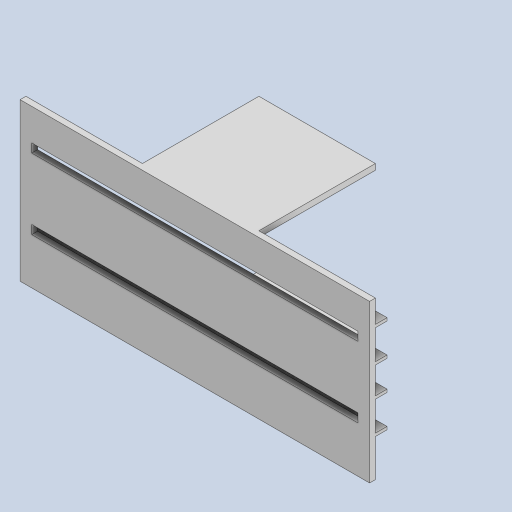
# Autodesk Inventor part: hand-box
Saved by Autodesk Inventor 2023 (Build 270158000, 158)
## iProperties
Created: 2024-11-28
Part Number: hand-box
Material: Generic
Document SubType Name: Modeling
Designer: kiyo
Density: 1 g/cm^3
Appearance: Default
Author: kiyo
Autodesk Inventor part; units mm, degrees
ref_plane "YZ Plane" through (0, 0, 0) normal (1, 0, 0) x (0, 1, 0)
ref_plane "XZ Plane" through (0, 0, 0) normal (0, 1, 0) x (-1, 0, 0)
ref_plane "XY Plane" through (0, 0, 0) normal (0, 0, 1) x (1, 0, 0)
sketch "スケッチ1" plane through (0, 0, 0) normal (1, 0, 0) x (0, 1, 0)
  line L0 (60, -16.042) -> (-60, -16.042)
  line L1 (-60, -16.042) -> (-60, 16.042)
  line L2 (-60, 16.042) -> (60, 16.042)
  line L3 (60, 16.042) -> (60, -16.042)
  line L4 (60, -16.042) -> (-60, 16.042) construction
  line L5 (-60, -16.042) -> (60, 16.042) construction
  line L6 (-56, 13.625) -> (56, 13.625)
  line L7 (56, 13.625) -> (56, 10.625)
  line L8 (56, 10.625) -> (-56, 10.625)
  line L9 (-56, 10.625) -> (-56, 13.625)
  line L10 (-56, -10.625) -> (56, -10.625)
  line L11 (56, -10.625) -> (56, -13.625)
  line L12 (56, -13.625) -> (-56, -13.625)
  line L13 (-56, -13.625) -> (-56, -10.625)
  line L14 (60, -16.042) -> (-60, -16.042)
  line L15 (-60, -16.042) -> (-60, -29.5)
  line L16 (-60, -29.5) -> (60, -29.5)
  line L17 (60, -29.5) -> (60, -16.042)
  line L18 (-60, 16.042) -> (60, 16.042)
  line L19 (60, 16.042) -> (60, 24.5)
  line L20 (60, 24.5) -> (-60, 24.5)
  line L21 (-60, 24.5) -> (-60, 16.042)
  point P0 (0, 0)
  point P1 (0, 0)
  point P2 (56, 12.125)
  point P3 (56, -12.125)
  point P4 (0, 0)
  dimension "d1" = 120
  dimension "d3" = 12.125
  dimension "d6" = 3
  dimension "d11" = 12.125
  dimension "d15" = 2.417
  dimension "d26" = 4
  dimension "d27" = 4
  dimension "d41" = 29.5
  dimension "d53" = 54
  constraints: 44 end point, 10 parallel, 6 midpoint, 5 horizontal, 5 perpendicular, 3 collinear, 2 point on line
  measures "d1" distance of L1.end L2.end
  measures "d3" vertical distance of point (56, -12.125) point (0, 0)
  measures "d6" distance of L8.end L6.start
  measures "d11" vertical distance of point (0, 0) point (56, 12.125)
  measures "d15" distance between parallel lines of L2 L6
  measures "d26" distance between parallel lines of L3 L7
  measures "d27" distance between parallel lines of L1 L9
  measures "d41" distance from line of L16 point (0, 0)
  measures "d53" distance between parallel lines of L16 L20
extrude "押し出し1" add sketch "スケッチ1" along normal blind 2
sketch "スケッチ3" plane through (0, 0, 0) normal (-1, 0, 0) x (0, 0, 1)
  line L0 (-29.5, 60) -> (24.5, 60) projected
  line L1 (5.575, 60) -> (4.575, 60)
  line L2 (4.575, 60) -> (4.575, 7)
  line L3 (4.575, 7) -> (5.575, 7)
  line L4 (5.575, 7) -> (5.575, 60)
  line L5 (16.675, 60) -> (15.675, 60)
  line L6 (15.675, 60) -> (15.675, 0)
  line L7 (15.675, 0) -> (16.675, 0)
  line L8 (16.675, 0) -> (16.675, 60)
  line L9 (0, 0) -> (4.575, 0)
  line L10 (0, 0) -> (0, 19.0491)
  line L11 (5.575, -60) -> (4.575, -60)
  line L12 (4.575, -60) -> (4.575, -7)
  line L13 (4.575, -7) -> (5.575, -7)
  line L14 (5.575, -7) -> (5.575, -60)
  line L15 (16.675, -60) -> (15.675, -60)
  line L16 (15.675, -60) -> (15.675, 0)
  line L17 (16.675, 0) -> (16.675, -60)
  line L18 (-5.575, 60) -> (-4.575, 60)
  line L19 (-4.575, 60) -> (-4.575, 7)
  line L20 (-4.575, 7) -> (-5.575, 7)
  line L21 (-5.575, 7) -> (-5.575, 60)
  line L22 (-16.675, 60) -> (-15.675, 60)
  line L23 (-15.675, 60) -> (-15.675, 0)
  line L24 (-15.675, 0) -> (-16.675, 0)
  line L25 (-16.675, 0) -> (-16.675, 60)
  line L26 (-5.575, -60) -> (-4.575, -60)
  line L27 (-4.575, -60) -> (-4.575, -7)
  line L28 (-4.575, -7) -> (-5.575, -7)
  line L29 (-5.575, -7) -> (-5.575, -60)
  line L30 (-16.675, -60) -> (-15.675, -60)
  line L31 (-15.675, -60) -> (-15.675, 0)
  line L32 (-16.675, 0) -> (-16.675, -60)
  point P0 (-15.675, 60)
  point P1 (-16.675, 60)
  point P2 (15.675, 60)
  point P3 (0, 9.5245)
  dimension "d31" = 1
  dimension "d33" = 1
  dimension "d34" = 60
  dimension "d35" = 10.1
  dimension "d36" = 7
  dimension "d61" = 5.575
  constraints: 64 end point, 20 symmetric about line, 4 parallel, 3 horizontal, 2 perpendicular, 1 midpoint, 1 point on line, 1 vertical
  measures "d31" distance of L2.end L3.end
  measures "d33" distance of L6.end L7.end
  measures "d34" distance of L7.end L5.start
  measures "d35" distance between parallel lines of L6 L4
  measures "d36" distance from line of L9.start L3
  measures "d61" distance between parallel lines of L4 L10
extrude "押し出し4" add sketch "スケッチ3" along normal blind 4
sketch "スケッチ5" plane through (0, 0, 0) normal (-1, 0, 0) x (0, 0, 1)
  line L0 (-29.5, -60) -> (-29.5, 60) projected
  line L1 (-29.5, 20) -> (-27.5, 20)
  line L2 (-27.5, 20) -> (-27.5, -20)
  line L3 (-27.5, -20) -> (-29.5, -20)
  line L4 (-29.5, -20) -> (-29.5, 60)
  line L5 (24.5, 60) -> (24.5, -60) projected
  line L6 (24.5, 20) -> (22.5, 20)
  line L7 (22.5, 20) -> (22.5, -20)
  line L8 (22.5, -20) -> (24.5, -20)
  line L9 (24.5, -20) -> (24.5, 20)
  point P0 (0, 0)
  point P1 (-29.5, -20)
  dimension "d42" = 2
  dimension "d55" = 20
  dimension "d56" = 20
  dimension "d57" = 2
  constraints: 16 end point, 4 parallel, 2 collinear, 2 horizontal, 2 perpendicular, 2 point on line
  measures "d42" distance between parallel lines of L0 L2
  measures "d55" distance from line of point (0, 0) L3
  measures "d56" distance from line of L1 point (0, 0)
  measures "d57" distance of L7.end L8.end
extrude "押し出し5" add sketch "スケッチ5" along normal blind 40
sketch "スケッチ6" plane through (2, -60, -29.5) normal (0, 0, -1) x (-1, 0, 0)
  circle A0 centre (20.75, 67) radius 1.6
  circle A1 centre (20.75, 53) radius 1.6
  line L0 (0, 0) -> (0, 120) projected
  point P0 (2, 60)
  point P1 (0, 60)
  dimension "d45" = 3.2
  dimension "d46" = 3.2
  dimension "d47" = 14
  dimension "d48" = 7
  dimension "d49" = 20.75
  dimension "d50" = 20.75
  constraints: 2 centre point, 1 midpoint
  measures "d45" diameter of A0
  measures "d46" diameter of A1
  measures "d47" distance of A0.centre A1.centre
  measures "d48" vertical distance of point (0, 60) A0.centre
  measures "d49" distance from line of L0 A0.centre
  measures "d50" distance from line of L0 A1.centre
extrude "押し出し6" cut sketch "スケッチ6" against normal blind 2
equation "\"d55\" = d56"
equation "\"d2\" = 0.25 * d0"
equation "\"d0\" = 30"
